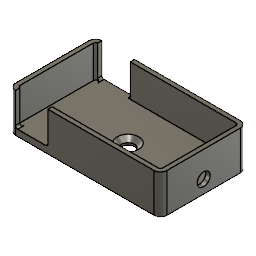
Sensor Case (Autodesk Fusion 360 design; units mm, degrees)
Autodesk Fusion 360 part; units mm, degrees
note: some values were not read from the file. Chosen so that the rebuilt part matches the saved one: which face or edge a step refers to.
sketch "Sketch1" plane through (0, 0, 0) normal (0, 1, 0) x (1, 0, 0)
  line L0 (-35, 20) -> (35, 20)
  line L1 (35, 20) -> (35, -20)
  line L2 (35, -20) -> (-35, -20)
  line L3 (-35, -20) -> (-35, 20)
  line L4 (-35, 20) -> (35, -20) construction
  dimension "d82" = 70
  dimension "d83" = 40
  constraint horizontal L0
  constraint vertical L1
  constraint horizontal L2
  constraint vertical L3
  constraint midpoint origin L4
  measures "d82" distance of L0.start L0.end
  measures "d83" distance of L0.start L2.end
extrude "Extrude1" add sketch "Sketch1" along normal blind 3
sketch "Sketch2" plane through (0, 3, 0) normal (0, 1, 0) x (-1, 0, 0)
  line L0 (35, 20) -> (-35, 20)
  line L1 (-35, 20) -> (-35, -20)
  line L2 (-35, -20) -> (35, -20)
  line L3 (35, -20) -> (35, 20)
  line L4 (33, 18) -> (-33, 18)
  line L5 (-33, 18) -> (-33, -18)
  line L6 (-33, -18) -> (33, -18)
  line L7 (33, -18) -> (33, 18)
  dimension "d86" = -2
extrude "Extrude2" add sketch "Sketch2" along normal blind 15
fillet "Fillet1" radius 1 4 edges at (-33, 10.5, -18) (33, 10.5, -18) (33, 10.5, 18) (-33, 10.5, 18)
fillet "Fillet2" radius 3 4 edges at (35, 9, -20) (-35, 9, -20) (35, 9, 20) (-35, 9, 20)
sketch "Sketch3" plane through (0, 0, 0) normal (0, 0, 1) x (1, 0, 0)
  line L0 (-32, 18) -> (-17, 18)
  line L1 (-17, 18) -> (-17, 3)
  line L2 (-17, 3) -> (-32, 3)
  line L3 (-32, 3) -> (-32, 18)
  dimension "d91" = 3
  dimension "d92" = 15
  dimension "d93" = 32
  dimension "d94" = 15
  constraint horizontal L0
  constraint vertical L1
  constraint horizontal L2
  constraint vertical L3
  measures "d91" distance of origin L2
  measures "d92" distance of L0.start L0.end
  measures "d93" distance of origin L3
  measures "d94" distance of L0.start L2.end
extrude "Extrude3" cut sketch "Sketch3" along normal mid plane 54
sketch "Sketch4" plane through (35, 0, 0) normal (1, 0, 0) x (0, 0, -1)
  line L0 (-17, 18) -> (-17, 0)
  line L1 (-17, 0) -> (17, 0)
  line L2 (17, 0) -> (17, 18)
  line L3 (17, 18) -> (-17, 18)
  circle A0 centre (0, 6) radius 3
  line L4 (0, 6) -> (0, 0) construction
  dimension "d97" = 6
  dimension "d98" = 6
  constraint coincident A0.centre L4.start
  constraint coincident L4.end origin
  constraint vertical L4
  measures "d97" diameter of A0
  measures "d98" distance of A0.centre L4.end
extrude "Extrude4" cut sketch "Sketch4" against normal blind 3 contours A0
fillet "Fillet3" radius 1 4 edges at (-32, 3, -19) (-32, 3, 19) (-17, 3, -19) (-17, 3, 19)
sketch "Sketch5" plane through (0, 3, 0) normal (0, 1, 0) x (-1, 0, 0)
  line L0 (18, 20) -> (18, 18)
  line L1 (18, 18) -> (-32, 18)
  arc A0 (-32, 18) -> (-33, 17) centre (-32, 17) ccw
  line L2 (-33, 17) -> (-33, 0)
  line L3 (-33, 0) -> (-33, -17)
  arc A1 (-33, -17) -> (-32, -18) centre (-32, -17) ccw
  line L4 (-32, -18) -> (18, -18)
  line L5 (18, -18) -> (18, -20)
  line L6 (18, -20) -> (31, -20)
  line L7 (31, -20) -> (31, -17)
  arc A2 (31, -17) -> (33, -17) centre (32, -17) ccw
  line L8 (33, -17) -> (33, 17)
  arc A3 (33, 17) -> (31, 17) centre (32, 17) ccw
  line L9 (31, 17) -> (31, 20)
  line L10 (31, 20) -> (18, 20)
  circle A4 centre (0, 0) radius 3
  dimension "d102" = 6
  constraint coincident A4.centre origin
  measures "d102" diameter of A4
extrude "Extrude5" cut sketch "Sketch5" against normal blind 3 contours A4
chamfer "Chamfer1" distance 2 angle 45 1 edges at (2.797, 3, 1.0848)
